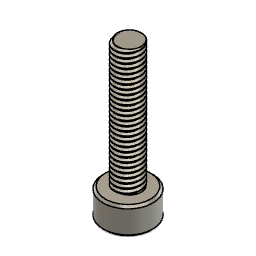
leg-test-stand-v4 (Autodesk Fusion 360 archive; units mm, degrees)
design "Cub Head Screw HEX (M3, 14mm)"
Autodesk Fusion 360 part; units mm, degrees
(part 1 of 2)
sketch "Sketch1" plane through (0, 0, 0) normal (0, 1, 0) x (1, 0, 0)
  circle A0 centre (0, 0) radius 1.5
  circle A1 centre (0, 0) radius 2.75
  line L0 (0.7217, -1.25) -> (1.4434, 0)
  line L1 (1.4434, 0) -> (0.7217, 1.25)
  line L2 (0.7217, 1.25) -> (-0.7217, 1.25)
  line L3 (-0.7217, 1.25) -> (-1.4434, 0)
  line L4 (-1.4434, 0) -> (-0.7217, -1.25)
  line L5 (-0.7217, -1.25) -> (0.7217, -1.25)
  dimension "d6" = 3
  dimension "d7" = 5.5
  dimension "d8" = 1.25
  constraint coincident A0.centre A1.centre
  constraint concentric A0 A1
  measures "d6" diameter of A0
  measures "d7" diameter of A1
  measures "d8" distance of A0.centre L5
extrude "Extrude1" add sketch "Sketch1" along normal blind 3 contours A0 | A1 | L0 L1 L2 L3 L4 L5
extrude "Extrude2" add sketch "Sketch1" along normal blind 17 contours A0 | L0 L1 L2 L3 L4 L5
extrude "Extrude3" cut sketch "Sketch1" along normal blind 1.5 contours L0 L1 L2 L3 L4 L5
thread "Thread1" "ISO Metric profile 3.0 M3x0.5 6g" major diameter 2.927 minor diameter 2.3555 pitch 0.5 angle 60 modelled right hand crest width 0.0713 on face at (1.4925, 7.6667, -0.1494) crest through (1.4635, 2.875, 0)
chamfer "Chamfer2" distance 0.25 angle 45 1 edges at (-2.5639, 3, 0.9944) 1 faces at (-0.0685, 0, 1.7474)
equation "Thread_Diameter = 3 mm"
equation "Thread_Length = 14 mm"
equation "Head_Diameter = 5.5 mm"
equation "Head_Height = 3 mm"
equation "Hex_Size = 2.5 mm"
equation "d6 = Thread_Diameter"
equation "d7 = Head_Diameter"
equation "d8 = Hex_Size / 2"
equation "d9 = Head_Height"
equation "d11 = Head_Height + Thread_Length"
equation "d13 = Head_Height / 2"

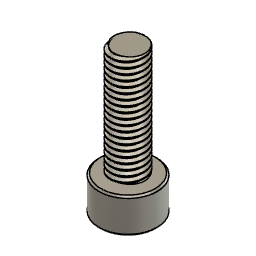
design "Cub Head Screw HEX (M5, 16mm)"
Autodesk Fusion 360 part; units mm, degrees
sketch "Sketch1" plane through (0, 0, 0) normal (0, 1, 0) x (1, 0, 0)
  circle A0 centre (0, 0) radius 2.5
  circle A1 centre (0, 0) radius 4.2
  line L0 (1.1547, -2) -> (2.3094, 0)
  line L1 (2.3094, 0) -> (1.1547, 2)
  line L2 (1.1547, 2) -> (-1.1547, 2)
  line L3 (-1.1547, 2) -> (-2.3094, 0)
  line L4 (-2.3094, 0) -> (-1.1547, -2)
  line L5 (-1.1547, -2) -> (1.1547, -2)
  dimension "d6" = 5
  dimension "d7" = 8.4
  dimension "d8" = 2
  constraint coincident A0.centre A1.centre
  constraint concentric A0 A1
  measures "d6" diameter of A0
  measures "d7" diameter of A1
  measures "d8" distance of A0.centre L5
extrude "Extrude1" add sketch "Sketch1" along normal blind 5 contours A0 | A1 | L0 L1 L2 L3 L4 L5
extrude "Extrude2" add sketch "Sketch1" along normal blind 21 contours A0 | L0 L1 L2 L3 L4 L5
extrude "Extrude3" cut sketch "Sketch1" along normal blind 2.5 contours L0 L1 L2 L3 L4 L5
thread "Thread1" "ISO Metric profile 5.0 M5x0.8 6g" major diameter 4.901 minor diameter 3.9895 pitch 0.8 angle 60 modelled right hand crest width 0.1157 on face at (2.4876, 10.3333, -0.2489) crest through (2.4505, 4.8, 0)
chamfer "Chamfer2" distance 0.25 angle 45 1 edges at (-3.9158, 5, 1.5188) 1 faces at (-0.1046, 0, 2.7294)
equation "Thread_Diameter = 5 mm"
equation "Thread_Length = 16 mm"
equation "Head_Diameter = 8.4 mm"
equation "Head_Height = 5 mm"
equation "Hex_Size = 4 mm"
equation "d6 = Thread_Diameter"
equation "d7 = Head_Diameter"
equation "d8 = Hex_Size / 2"
equation "d9 = Head_Height"
equation "d11 = Head_Height + Thread_Length"
equation "d13 = Head_Height / 2"

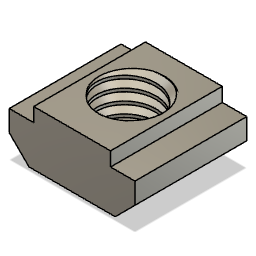
design "T-Nut (M5)"
Autodesk Fusion 360 part; units mm, degrees
sketch "Sketch1" plane through (0, 0, 0) normal (0, 0, 1) x (1, 0, 0)
  line L0 (0, 0) -> (4.5, 0)
  line L1 (4.5, 0) -> (4.5, -1.5)
  line L2 (4.5, -1.5) -> (3.0858, -2.9142)
  line L3 (4.5, -1.5) -> (6.5, -1.5) construction
  line L4 (0, 0) -> (-4.5, 0)
  line L5 (-4.5, 0) -> (-4.5, -1.5)
  line L6 (-4.5, -1.5) -> (-3.0858, -2.9142)
  line L7 (-3.0858, -2.9142) -> (3.0858, -2.9142)
  line L8 (0, 0) -> (2.75, 0)
  line L9 (2.75, 0) -> (2.75, 1)
  line L10 (0, 0) -> (-2.75, 0)
  line L11 (-2.75, 0) -> (-2.75, 1)
  line L12 (-2.75, 1) -> (2.75, 1)
  dimension "d1" = 4.5
  dimension "d2" = 1.5
  dimension "d3" = 135
  dimension "d4" = 2
  dimension "d5" = 135
  dimension "d6" = 4.5
  dimension "d7" = 1.5
  dimension "d8" = 2
  dimension "d9" = 2.75
  dimension "d10" = 1
  dimension "d11" = 2.75
  dimension "d12" = 1
  constraint coincident L0.start L4.start
  constraint horizontal L0
  constraint perpendicular L0 L1
  constraint horizontal L3
  constraint parallel L0 L4
  constraint perpendicular L0 L5
  constraint parallel L0 L8
  constraint perpendicular L8 L9
  constraint parallel L4 L10
  constraint perpendicular L4 L11
  measures "d1" distance of L0.start L0.end
  measures "d2" distance of L0.end L1.end
  measures "d3" angle of L2 L3
  measures "d4" distance of L1.end L2.end
  measures "d5" angle of L5 L6
  measures "d6" distance of L0.start L4.end
  measures "d7" distance of L4.end L5.end
  measures "d8" distance of L5.end L6.end
  measures "d9" distance of L0.start L8.end
  measures "d10" distance of L8.end L9.end
  measures "d11" distance of L0.start L10.end
  measures "d12" distance of L10.end L11.end
extrude "Extrude1" add sketch "Sketch1" along normal mid plane 8
sketch "Sketch2" plane through (0, 1, 0) normal (0, 1, 0) x (-1, 0, 0)
  line L0 (2.75, -4) -> (2.75, 4)
  line L1 (2.75, 4) -> (-2.75, 4)
  line L2 (-2.75, 4) -> (-2.75, -4)
  line L3 (-2.75, -4) -> (2.75, -4)
  circle A0 centre (0, 0) radius 2.5
  dimension "d15" = 5
  constraint coincident A0.centre origin
  measures "d15" diameter of A0
extrude "Extrude2" cut sketch "Sketch2" against normal blind 3.9142 contours A0
thread "Thread1" "ISO Metric profile 5.0 M5x0.8 6H" major diameter 5.12 minor diameter 4.234 pitch 0.8 angle 60 modelled right hand crest width 0.2219 on face at (-2.4876, -1.6095, -0.2489) crest through (-2.117, 0.8, 0)
equation "d5 = d3"
equation "d6 = d1"
equation "d7 = d2"
equation "d8 = d4"
equation "d11 = d9"
equation "d12 = d10"

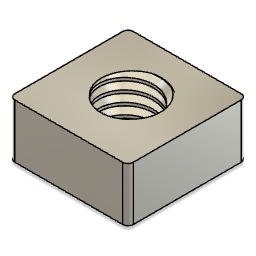
design "Square-Nut (M3)"
Autodesk Fusion 360 part; units mm, degrees
sketch "Sketch1" plane through (0, 0, 0) normal (0, 1, 0) x (1, 0, 0)
  line L0 (2.5, -2.75) -> (-2.5, -2.75)
  line L1 (-2.75, -2.5) -> (-2.75, 2.5)
  line L2 (-2.5, 2.75) -> (2.5, 2.75)
  line L3 (2.75, 2.5) -> (2.75, -2.5)
  line L4 (2.75, -2.75) -> (-2.75, 2.75) construction
  line L5 (-2.75, -2.75) -> (2.75, 2.75) construction
  circle A0 centre (0, 0) radius 1.5
  arc A1 (-2.5, 2.75) -> (-2.75, 2.5) centre (-2.5, 2.5) ccw
  arc A2 (2.75, 2.5) -> (2.5, 2.75) centre (2.5, 2.5) ccw
  arc A3 (2.5, -2.75) -> (2.75, -2.5) centre (2.5, -2.5) ccw
  arc A4 (-2.75, -2.5) -> (-2.5, -2.75) centre (-2.5, -2.5) ccw
  dimension "d1" = 5.5
  dimension "d2" = 5.5
  dimension "d3" = 3
  dimension "d4" = 0.25
  constraint horizontal L0
  constraint perpendicular L0 L1
  constraint parallel L0 L2
  constraint parallel L1 L3
  constraint coincident L4 A0.centre
  constraint coincident L5 A0.centre
  constraint coincident A0.centre origin
  constraint coincident L4.end L1
  constraint coincident L4.end L2
  constraint tangent L1 A1
  constraint tangent L2 A1
  constraint coincident L5.end L2
  constraint coincident L5.end L3
  constraint tangent L2 A2
  constraint tangent L3 A2
  constraint equal A1 A2
  constraint coincident L4.start L3
  constraint coincident L4.start L0
  constraint tangent L3 A3
  constraint tangent L0 A3
  constraint equal A1 A3
  constraint coincident L5.start L0
  constraint coincident L5.start L1
  constraint tangent L0 A4
  constraint tangent L1 A4
  constraint equal A1 A4
  measures "d1" distance of L4.end L5.end
  measures "d2" distance of L5.start L4.end
  measures "d3" diameter of A0
  measures "d4" radius of A1
extrude "Extrude1" add sketch "Sketch1" along normal blind 2.5
thread "Thread1" "ISO Metric profile 3.0 M3x0.5 6H" major diameter 3.086 minor diameter 2.529 pitch 0.5 angle 60 modelled right hand crest width 0.1368 on face at (1.4981, 1.6667, 0.0748) crest through (1.2645, 0.125, 0)
equation "d2 = d1"

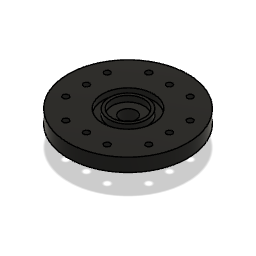
design "MG996R-servo horn"
Autodesk Fusion 360 part; units mm, degrees
sketch "Sketch1" plane through (0, 0, 0) normal (0, 1, 0) x (1, 0, 0)
  circle A0 centre (0, 0) radius 10.35
  circle A1 centre (0, 0) radius 4.4
  circle A2 centre (0, 0) radius 2.8
  circle A3 centre (0, 0) radius 3.3
  circle A4 centre (0, 0) radius 1.4
  circle A5 centre (0, 0) radius 2.6
  circle A6 centre (0, 7.2) radius 0.5
  circle A7 centre (-3.6, 7.2) radius 0.5
  circle A8 centre (3.6, 7.2) radius 0.5
  circle A9 centre (-7.2, 3.6) radius 0.5
  circle A10 centre (-7.2, 0) radius 0.5
  circle A11 centre (-7.2, -3.6) radius 0.5
  circle A12 centre (-3.6, -7.2) radius 0.5
  circle A13 centre (0, -7.2) radius 0.5
  circle A14 centre (3.6, -7.2) radius 0.5
  circle A15 centre (7.2, -3.6) radius 0.5
  circle A16 centre (7.2, 0) radius 0.5
  circle A17 centre (7.2, 3.6) radius 0.5
  dimension "d1" = 20.7
  dimension "d2" = 8.8
  dimension "d3" = 5.6
  dimension "d4" = 6.6
  dimension "d5" = 2.8
  dimension "d6" = 5.2
  dimension "d7" = 1
  dimension "d8" = 7.2
  dimension "d11" = 3.6
  dimension "d12" = 0
  dimension "d14" = 360
  constraint coincident A0.centre A1.centre
  constraint concentric A0 A1
  constraint concentric A0 A2
  constraint concentric A1 A3
  constraint concentric A1 A5
  measures "d1" diameter of A0
  measures "d2" diameter of A1
  measures "d3" diameter of A2
  measures "d4" diameter of A3
  measures "d5" diameter of A4
  measures "d6" diameter of A5
  measures "d7" diameter of A6
  measures "d8" distance of A0.centre A6.centre
extrude "Extrude1" add sketch "Sketch1" against normal blind 3.55 contours A1 | A2 | A3
extrude "Extrude4" add sketch "Sketch1" against normal blind 0.55 contours A5
extrude "Extrude2" add sketch "Sketch1" along normal blind 2.3 contours A0 | A1 | A2 | A3 | A5
extrude "Extrude3" cut sketch "Sketch1" against normal blind 1 from surface at 2.3 contours A1 | A2 | A5
equation "d8 = ( 14.4 / 2 ) * 1 mm"

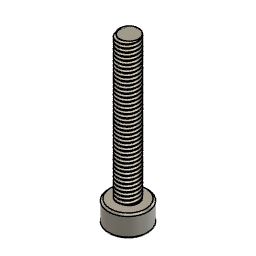
design "Cub Head Screw HEX (M3, 20mm)"
Autodesk Fusion 360 part; units mm, degrees
sketch "Sketch1" plane through (0, 0, 0) normal (0, 1, 0) x (1, 0, 0)
  circle A0 centre (0, 0) radius 1.5
  circle A1 centre (0, 0) radius 2.75
  line L0 (0.7217, -1.25) -> (1.4434, 0)
  line L1 (1.4434, 0) -> (0.7217, 1.25)
  line L2 (0.7217, 1.25) -> (-0.7217, 1.25)
  line L3 (-0.7217, 1.25) -> (-1.4434, 0)
  line L4 (-1.4434, 0) -> (-0.7217, -1.25)
  line L5 (-0.7217, -1.25) -> (0.7217, -1.25)
  dimension "d6" = 3
  dimension "d7" = 5.5
  dimension "d8" = 1.25
  constraint coincident A0.centre A1.centre
  constraint concentric A0 A1
  measures "d6" diameter of A0
  measures "d7" diameter of A1
  measures "d8" distance of A0.centre L5
extrude "Extrude1" add sketch "Sketch1" along normal blind 3 contours A0 | A1 | L0 L1 L2 L3 L4 L5
extrude "Extrude2" add sketch "Sketch1" along normal blind 23 contours A0 | L0 L1 L2 L3 L4 L5
extrude "Extrude3" cut sketch "Sketch1" along normal blind 1.5 contours L0 L1 L2 L3 L4 L5
thread "Thread1" "ISO Metric profile 3.0 M3x0.5 6g" major diameter 2.927 minor diameter 2.3555 pitch 0.5 angle 60 modelled right hand crest width 0.0713 on face at (1.4925, 9.6667, -0.1494) crest through (1.4635, 2.875, 0)
chamfer "Chamfer2" distance 0.25 angle 45 1 edges at (-2.5639, 3, 0.9944) 1 faces at (-0.0685, 0, 1.7474)
equation "Thread_Diameter = 3 mm"
equation "Thread_Length = 20 mm"
equation "Head_Diameter = 5.5 mm"
equation "Head_Height = 3 mm"
equation "Hex_Size = 2.5 mm"
equation "d6 = Thread_Diameter"
equation "d7 = Head_Diameter"
equation "d8 = Hex_Size / 2"
equation "d9 = Head_Height"
equation "d11 = Head_Height + Thread_Length"
equation "d13 = Head_Height / 2"

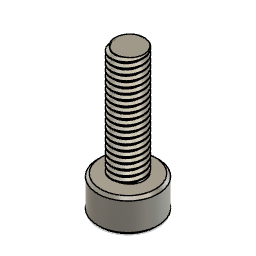
design "Cub Head Screw HEX (M3, 10mm)"
Autodesk Fusion 360 part; units mm, degrees
sketch "Sketch1" plane through (0, 0, 0) normal (0, 1, 0) x (1, 0, 0)
  circle A0 centre (0, 0) radius 1.5
  circle A1 centre (0, 0) radius 2.75
  line L0 (0.7217, -1.25) -> (1.4434, 0)
  line L1 (1.4434, 0) -> (0.7217, 1.25)
  line L2 (0.7217, 1.25) -> (-0.7217, 1.25)
  line L3 (-0.7217, 1.25) -> (-1.4434, 0)
  line L4 (-1.4434, 0) -> (-0.7217, -1.25)
  line L5 (-0.7217, -1.25) -> (0.7217, -1.25)
  dimension "d6" = 3
  dimension "d7" = 5.5
  dimension "d8" = 1.25
  constraint coincident A0.centre A1.centre
  constraint concentric A0 A1
  measures "d6" diameter of A0
  measures "d7" diameter of A1
  measures "d8" distance of A0.centre L5
extrude "Extrude1" add sketch "Sketch1" along normal blind 3 contours A0 | A1 | L0 L1 L2 L3 L4 L5
extrude "Extrude2" add sketch "Sketch1" along normal blind 13 contours A0 | L0 L1 L2 L3 L4 L5
extrude "Extrude3" cut sketch "Sketch1" along normal blind 1.5 contours L0 L1 L2 L3 L4 L5
thread "Thread1" "ISO Metric profile 3.0 M3x0.5 6g" major diameter 2.927 minor diameter 2.3555 pitch 0.5 angle 60 modelled right hand crest width 0.0713 on face at (1.4925, 6.3333, -0.1494) crest through (1.4635, 2.875, 0)
chamfer "Chamfer2" distance 0.25 angle 45 1 edges at (-2.5639, 3, 0.9944) 1 faces at (-0.0685, 0, 1.7474)
equation "Thread_Diameter = 3 mm"
equation "Thread_Length = 10 mm"
equation "Head_Diameter = 5.5 mm"
equation "Head_Height = 3 mm"
equation "Hex_Size = 2.5 mm"
equation "d6 = Thread_Diameter"
equation "d7 = Head_Diameter"
equation "d8 = Hex_Size / 2"
equation "d9 = Head_Height"
equation "d11 = Head_Height + Thread_Length"
equation "d13 = Head_Height / 2"

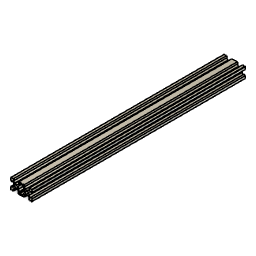
design "Extrusions-2040 (400mm)"
Autodesk Fusion 360 part; units mm, degrees
sketch "Skizze1" plane through (0, 0, 0) normal (0, 0, 1) x (1, 0, 0)
  line L0 (0, 0) -> (20, 0)
  line L1 (20, 0) -> (20, 20)
  line L2 (20, 20) -> (0, 20)
  line L3 (0, 20) -> (0, 0)
  circle A0 centre (10, 10) radius 2.5
  line L4 (0, 0) -> (6.8, 0)
  line L5 (6.8, 0) -> (13.2, 0)
  line L6 (6.8, 0) -> (13.2, 0)
  line L7 (13.2, 0) -> (13.2, 1.8)
  line L8 (13.2, 1.8) -> (6.8, 1.8)
  line L9 (6.8, 1.8) -> (6.8, 0)
  line L10 (0, 0) -> (0, 6.8)
  line L11 (0, 20) -> (6.8, 20)
  line L12 (20, 0) -> (20, 6.8)
  line L13 (0, 6.8) -> (1.8, 6.8)
  line L14 (1.8, 6.8) -> (1.8, 13.2)
  line L15 (1.8, 13.2) -> (0, 13.2)
  line L16 (0, 13.2) -> (0, 6.8)
  line L17 (6.8, 20) -> (13.2, 20)
  line L18 (13.2, 20) -> (13.2, 18.2)
  line L19 (13.2, 18.2) -> (6.8, 18.2)
  line L20 (6.8, 18.2) -> (6.8, 20)
  line L21 (20, 6.8) -> (18.2, 6.8)
  line L22 (18.2, 6.8) -> (18.2, 13.2)
  line L23 (18.2, 13.2) -> (20, 13.2)
  line L24 (20, 13.2) -> (20, 6.8)
  line L25 (10, 1.8) -> (15, 1.8)
  line L26 (15, 1.8) -> (15, 3.6)
  line L27 (15, 3.6) -> (10, 3.6)
  line L28 (10, 3.6) -> (10, 1.8)
  line L29 (15, 1.8) -> (5, 1.8)
  line L30 (5, 1.8) -> (5, 3.6)
  line L31 (5, 3.6) -> (15, 3.6)
  line L32 (15, 3.6) -> (15, 1.8)
  line L33 (10, 18.2) -> (15, 18.2)
  line L34 (15, 18.2) -> (15, 16.4)
  line L35 (15, 16.4) -> (10, 16.4)
  line L36 (10, 16.4) -> (10, 18.2)
  line L37 (15, 16.4) -> (5, 16.4)
  line L38 (5, 16.4) -> (5, 18.2)
  line L39 (5, 18.2) -> (15, 18.2)
  line L40 (15, 18.2) -> (15, 16.4)
  line L41 (1.8, 10) -> (3.6, 10)
  line L42 (3.6, 10) -> (3.6, 5)
  line L43 (3.6, 5) -> (1.8, 5)
  line L44 (1.8, 5) -> (1.8, 10)
  line L45 (3.6, 5) -> (1.8, 5)
  line L46 (1.8, 5) -> (1.8, 15)
  line L47 (1.8, 15) -> (3.6, 15)
  line L48 (3.6, 15) -> (3.6, 5)
  line L49 (18.2, 10) -> (16.4, 10)
  line L50 (16.4, 10) -> (16.4, 15)
  line L51 (16.4, 15) -> (18.2, 15)
  line L52 (18.2, 15) -> (18.2, 10)
  line L53 (16.4, 15) -> (18.2, 15)
  line L54 (18.2, 15) -> (18.2, 5)
  line L55 (18.2, 5) -> (16.4, 5)
  line L56 (16.4, 5) -> (16.4, 15)
  line L57 (6, 6) -> (14, 6)
  line L58 (14, 6) -> (14, 14)
  line L59 (14, 14) -> (6, 14)
  line L60 (6, 14) -> (6, 6)
  line L61 (5, 3.6) -> (7.4, 6)
  line L62 (5, 3.6) -> (8.3941, 3.6) construction
  line L63 (3.6, 5) -> (6, 7.4)
  line L64 (15, 3.6) -> (12.6, 6)
  line L65 (16.4, 5) -> (14, 7.4)
  line L66 (16.4, 15) -> (14, 12.6)
  line L67 (15, 16.4) -> (12.6, 14)
  line L68 (3.6, 15) -> (6, 12.6)
  line L69 (5, 16.4) -> (7.4, 14)
  line L70 (6.8, 1.8) -> (5, 0)
  line L71 (18.2, 5) -> (20.7456, 5) construction
  line L72 (18.2, 6.8) -> (20, 5)
  line L73 (18.2, 13.2) -> (20, 15)
  line L74 (18.2, 13.2) -> (20.7456, 13.2) construction
  line L75 (6.8, 18.2) -> (5, 20)
  line L76 (13.2, 18.2) -> (15, 20)
  line L77 (1.8, 13.2) -> (0, 15)
  line L78 (1.8, 6.8) -> (0, 5)
  line L79 (13.2, 1.8) -> (15, 0)
  dimension "d1" = 5
  dimension "d2" = 6.8
  dimension "d3" = 6.4
  dimension "d4" = 1.8
  dimension "d5" = 6.8
  dimension "d6" = 6.8
  dimension "d7" = 6.8
  dimension "d8" = 1.8
  dimension "d9" = 6.4
  dimension "d10" = 1.8
  dimension "d11" = 1.8
  dimension "d12" = 5
  dimension "d13" = 1.8
  dimension "d14" = 10
  dimension "d15" = 1.8
  dimension "d16" = 1.8
  dimension "d17" = 10
  dimension "d18" = 1.8
  dimension "d19" = 10
  dimension "d20" = 45
  dimension "d22" = 45
  constraint horizontal L0
  constraint vertical L1
  constraint horizontal L2
  constraint vertical L3
  constraint coincident L0.start L3.end
  constraint perpendicular L3 L4
  constraint parallel L0 L5
  constraint horizontal L6
  constraint vertical L7
  constraint horizontal L8
  constraint vertical L9
  constraint perpendicular L4 L10
  constraint perpendicular L3 L11
  constraint perpendicular L11 L12
  constraint horizontal L13
  constraint vertical L14
  constraint horizontal L15
  constraint vertical L16
  constraint horizontal L17
  constraint vertical L18
  constraint horizontal L19
  constraint vertical L20
  constraint horizontal L21
  constraint vertical L22
  constraint horizontal L23
  constraint vertical L24
  constraint horizontal L25
  constraint vertical L26
  constraint horizontal L27
  constraint vertical L28
  constraint midpoint L8 L25.start
  constraint horizontal L29
  constraint vertical L30
  constraint horizontal L31
  constraint vertical L32
  constraint horizontal L33
  constraint vertical L34
  constraint horizontal L35
  constraint vertical L36
  constraint midpoint L19 L33.start
  constraint horizontal L37
  constraint vertical L38
  constraint horizontal L39
  constraint vertical L40
  constraint horizontal L41
  constraint vertical L42
  constraint horizontal L43
  constraint vertical L44
  constraint midpoint L14 L41.start
  constraint horizontal L45
  constraint vertical L46
  constraint horizontal L47
  constraint vertical L48
  constraint horizontal L49
  constraint vertical L50
  constraint horizontal L51
  constraint vertical L52
  constraint midpoint L22 L49.start
  constraint horizontal L53
  constraint vertical L54
  constraint horizontal L55
  constraint vertical L56
  constraint horizontal L57
  constraint vertical L58
  constraint horizontal L59
  constraint vertical L60
  constraint horizontal L62
  constraint coincident L57 L61.end
  constraint coincident L60 L63.end
  constraint parallel L61 L63
  constraint coincident L57 L64.end
  constraint perpendicular L63 L64
  constraint coincident L58 L65.end
  constraint parallel L64 L65
  constraint coincident L58 L66.end
  constraint perpendicular L65 L66
  constraint coincident L59 L67.end
  constraint parallel L66 L67
  constraint coincident L60 L68.end
  constraint perpendicular L67 L68
  constraint coincident L59 L69.end
  constraint parallel L68 L69
  constraint coincident L0 L70.end
  constraint horizontal L71
  constraint coincident L12 L72.end
  constraint horizontal L74
  constraint coincident L1 L73.end
  constraint coincident L2 L75.end
  constraint coincident L2 L76.end
  constraint perpendicular L75 L76
  constraint coincident L3 L77.end
  constraint perpendicular L76 L77
  constraint coincident L10 L78.end
  constraint coincident L0 L79.end
  measures "d1" diameter of A0
  measures "d2" distance of L0.start L4.end
  measures "d3" distance of L4.end L5.end
  measures "d4" distance of L4.end L8.end
  measures "d5" distance of L0.start L10.end
  measures "d6" distance of L2.end L11.end
  measures "d7" distance of L0.end L12.end
  measures "d8" distance of L10.end L13.end
  measures "d9" distance of L10.end L15.end
  measures "d10" distance of L11.end L19.end
  measures "d11" distance of L12.end L21.end
  measures "d12" distance of L25.start L25.end
  measures "d13" distance of L25.start L27.end
  measures "d14" distance of L25.end L29.end
  measures "d15" distance of L33.start L35.end
  measures "d16" distance of L41.start L41.end
  measures "d17" distance of L42.end L47.end
  measures "d18" distance of L49.start L49.end
  measures "d19" distance of L50.end L55.end
  measures "d20" angle of L61 L62
  measures "d22" angle of L73 L74
extrude "Extrusion1" add sketch "Skizze1" along normal mid plane 400 contours L0 L3 L4 L10 L29 L30 L43 L44 L45 L46 L57 L60 L61 L63 L70 L78 | L0 L1 L12 L25 L26 L29 L32 L54 L55 L57 L58 L64 L65 L72 L79 | L2 L3 L11 L38 L39 L46 L47 L59 L60 L68 L69 L75 L77 | L57 L58 L59 L60 | L1 L2 L33 L34 L39 L40 L51 L52 L53 L54 L58 L59 L66 L67 L73 L76 makes body 1
copy_body "Körper kopieren/einfügen1" bodies 1 makes body 2
move_body "Verschieben1" bodies 2 to x (1, 0, 0) y (0, 1, 0) z (0, 0, 1) at (25, 0, 0)
copy_body "Körper kopieren/einfügen2" bodies 2 makes body 3
move_body "Verschieben2" bodies 3 to x (1, 0, 0) y (0, 1, 0) z (0, 0, 1) at (0, 20, 0)
combine "Kombinieren1" operation add target body 2 tool bodies 3
sketch "Skizze2" plane through (0, 0, 200) normal (0, 0, 1) x (1, 0, 0)
  line L0 (40, 20) -> (38.2, 18.2)
  line L1 (38.2, 18.2) -> (40, 18.2)
  line L2 (40, 18.2) -> (40, 16.4)
  line L3 (40, 16.4) -> (37.6, 14)
  line L4 (37.6, 14) -> (32.4, 14)
  line L5 (32.4, 14) -> (30, 16.4)
  line L6 (30, 16.4) -> (30, 18.2)
  line L7 (30, 18.2) -> (31.8, 18.2)
  line L8 (31.8, 18.2) -> (30, 20)
  line L9 (30, 20) -> (31.8, 21.8)
  line L10 (31.8, 21.8) -> (30, 21.8)
  line L11 (30, 21.8) -> (30, 23.6)
  line L12 (30, 23.6) -> (32.4, 26)
  line L13 (32.4, 26) -> (37.6, 26)
  line L14 (37.6, 26) -> (40, 23.6)
  line L15 (40, 23.6) -> (40, 21.8)
  line L16 (40, 21.8) -> (38.2, 21.8)
  line L17 (38.2, 21.8) -> (40, 20)
  circle A0 centre (35, 30) radius 2.5
  circle A1 centre (35, 10) radius 2.5
  line L18 (45, 15) -> (45, 25)
  line L19 (45, 25) -> (43.2, 26.8)
  line L20 (43.2, 26.8) -> (43.2, 25)
  line L21 (43.2, 25) -> (41.4, 25)
  line L22 (41.4, 25) -> (39, 27.4)
  line L23 (39, 27.4) -> (39, 32.6)
  line L24 (39, 32.6) -> (41.4, 35)
  line L25 (41.4, 35) -> (43.2, 35)
  line L26 (43.2, 35) -> (43.2, 33.2)
  line L27 (43.2, 33.2) -> (45, 35)
  line L28 (45, 35) -> (45, 40)
  line L29 (45, 40) -> (40, 40)
  line L30 (40, 40) -> (38.2, 38.2)
  line L31 (38.2, 38.2) -> (40, 38.2)
  line L32 (40, 38.2) -> (40, 36.4)
  line L33 (40, 36.4) -> (37.6, 34)
  line L34 (37.6, 34) -> (32.4, 34)
  line L35 (32.4, 34) -> (30, 36.4)
  line L36 (30, 36.4) -> (30, 38.2)
  line L37 (30, 38.2) -> (31.8, 38.2)
  line L38 (31.8, 38.2) -> (30, 40)
  line L39 (30, 40) -> (25, 40)
  line L40 (25, 40) -> (25, 35)
  line L41 (25, 35) -> (26.8, 33.2)
  line L42 (26.8, 33.2) -> (26.8, 35)
  line L43 (26.8, 35) -> (28.6, 35)
  line L44 (28.6, 35) -> (31, 32.6)
  line L45 (31, 32.6) -> (31, 27.4)
  line L46 (31, 27.4) -> (28.6, 25)
  line L47 (28.6, 25) -> (26.8, 25)
  line L48 (26.8, 25) -> (26.8, 26.8)
  line L49 (26.8, 26.8) -> (25, 25)
  line L50 (25, 25) -> (25, 15)
  line L51 (25, 15) -> (26.8, 13.2)
  line L52 (26.8, 13.2) -> (26.8, 15)
  line L53 (26.8, 15) -> (28.6, 15)
  line L54 (28.6, 15) -> (31, 12.6)
  line L55 (31, 12.6) -> (31, 7.4)
  line L56 (31, 7.4) -> (28.6, 5)
  line L57 (28.6, 5) -> (26.8, 5)
  line L58 (26.8, 5) -> (26.8, 6.8)
  line L59 (26.8, 6.8) -> (25, 5)
  line L60 (25, 5) -> (25, 0)
  line L61 (25, 0) -> (30, 0)
  line L62 (30, 0) -> (31.8, 1.8)
  line L63 (31.8, 1.8) -> (30, 1.8)
  line L64 (30, 1.8) -> (30, 3.6)
  line L65 (30, 3.6) -> (32.4, 6)
  line L66 (32.4, 6) -> (37.6, 6)
  line L67 (37.6, 6) -> (40, 3.6)
  line L68 (40, 3.6) -> (40, 1.8)
  line L69 (40, 1.8) -> (38.2, 1.8)
  line L70 (38.2, 1.8) -> (40, 0)
  line L71 (40, 0) -> (45, 0)
  line L72 (45, 0) -> (45, 5)
  line L73 (45, 5) -> (43.2, 6.8)
  line L74 (43.2, 6.8) -> (43.2, 5)
  line L75 (43.2, 5) -> (41.4, 5)
  line L76 (41.4, 5) -> (39, 7.4)
  line L77 (39, 7.4) -> (39, 12.6)
  line L78 (39, 12.6) -> (41.4, 15)
  line L79 (41.4, 15) -> (43.2, 15)
  line L80 (43.2, 15) -> (43.2, 13.2)
  line L81 (43.2, 13.2) -> (45, 15)
  line L82 (26.8, 15) -> (26.8, 16.98)
  line L83 (26.8, 25) -> (26.8, 23.02)
  line L84 (26.8, 16.98) -> (28.8, 16.98)
  line L85 (28.8, 16.98) -> (28.8, 23.02)
  line L86 (28.8, 23.02) -> (26.8, 23.02)
  line L87 (26.8, 23.02) -> (26.8, 16.98)
  dimension "d25" = 1.98
  dimension "d26" = 1.98
  dimension "d27" = 2
  constraint coincident L52.end L53.start
  constraint perpendicular L53 L82
  constraint coincident L47.end L48.start
  constraint perpendicular L47 L83
  constraint horizontal L84
  constraint vertical L85
  constraint horizontal L86
  constraint vertical L87
  measures "d25" distance of L52.end L82.end
  measures "d26" distance of L47.end L83.end
  measures "d27" distance of L82.end L84.end
extrude "Extrusion2" cut sketch "Skizze2" against normal blind 126 contours L84 L85 L86 L87 bodies 2
sketch "Skizze3" plane through (0, 0, 200) normal (0, 0, 1) x (1, 0, 0)
  line L0 (28.8, 16.98) -> (26.8, 16.98)
  line L1 (26.8, 16.98) -> (26.8, 23.02)
  line L2 (26.8, 23.02) -> (28.8, 23.02)
  line L3 (28.8, 23.02) -> (28.8, 16.98)
  line L4 (40, 20) -> (38.2, 18.2)
  line L5 (38.2, 18.2) -> (40, 18.2)
  line L6 (40, 18.2) -> (40, 16.4)
  line L7 (40, 16.4) -> (37.6, 14)
  line L8 (37.6, 14) -> (32.4, 14)
  line L9 (32.4, 14) -> (30, 16.4)
  line L10 (30, 16.4) -> (30, 18.2)
  line L11 (30, 18.2) -> (31.8, 18.2)
  line L12 (31.8, 18.2) -> (30, 20)
  line L13 (30, 20) -> (31.8, 21.8)
  line L14 (31.8, 21.8) -> (30, 21.8)
  line L15 (30, 21.8) -> (30, 23.6)
  line L16 (30, 23.6) -> (32.4, 26)
  line L17 (32.4, 26) -> (37.6, 26)
  line L18 (37.6, 26) -> (40, 23.6)
  line L19 (40, 23.6) -> (40, 21.8)
  line L20 (40, 21.8) -> (38.2, 21.8)
  line L21 (38.2, 21.8) -> (40, 20)
  circle A0 centre (35, 30) radius 2.5
  circle A1 centre (35, 10) radius 2.5
  line L22 (45, 15) -> (45, 25)
  line L23 (45, 25) -> (43.2, 26.8)
  line L24 (43.2, 26.8) -> (43.2, 25)
  line L25 (43.2, 25) -> (41.4, 25)
  line L26 (41.4, 25) -> (39, 27.4)
  line L27 (39, 27.4) -> (39, 32.6)
  line L28 (39, 32.6) -> (41.4, 35)
  line L29 (41.4, 35) -> (43.2, 35)
  line L30 (43.2, 35) -> (43.2, 33.2)
  line L31 (43.2, 33.2) -> (45, 35)
  line L32 (45, 35) -> (45, 40)
  line L33 (45, 40) -> (40, 40)
  line L34 (40, 40) -> (38.2, 38.2)
  line L35 (38.2, 38.2) -> (40, 38.2)
  line L36 (40, 38.2) -> (40, 36.4)
  line L37 (40, 36.4) -> (37.6, 34)
  line L38 (37.6, 34) -> (32.4, 34)
  line L39 (32.4, 34) -> (30, 36.4)
  line L40 (30, 36.4) -> (30, 38.2)
  line L41 (30, 38.2) -> (31.8, 38.2)
  line L42 (31.8, 38.2) -> (30, 40)
  line L43 (30, 40) -> (25, 40)
  line L44 (25, 40) -> (25, 35)
  line L45 (25, 35) -> (26.8, 33.2)
  line L46 (26.8, 33.2) -> (26.8, 35)
  line L47 (26.8, 35) -> (28.6, 35)
  line L48 (28.6, 35) -> (31, 32.6)
  line L49 (31, 32.6) -> (31, 27.4)
  line L50 (31, 27.4) -> (28.6, 25)
  line L51 (28.6, 25) -> (26.8, 25)
  line L52 (26.8, 25) -> (26.8, 26.8)
  line L53 (26.8, 26.8) -> (25, 25)
  line L54 (25, 25) -> (25, 15)
  line L55 (25, 15) -> (26.8, 13.2)
  line L56 (26.8, 13.2) -> (26.8, 15)
  line L57 (26.8, 15) -> (28.6, 15)
  line L58 (28.6, 15) -> (31, 12.6)
  line L59 (31, 12.6) -> (31, 7.4)
  line L60 (31, 7.4) -> (28.6, 5)
  line L61 (28.6, 5) -> (26.8, 5)
  line L62 (26.8, 5) -> (26.8, 6.8)
  line L63 (26.8, 6.8) -> (25, 5)
  line L64 (25, 5) -> (25, 0)
  line L65 (25, 0) -> (30, 0)
  line L66 (30, 0) -> (31.8, 1.8)
  line L67 (31.8, 1.8) -> (30, 1.8)
  line L68 (30, 1.8) -> (30, 3.6)
  line L69 (30, 3.6) -> (32.4, 6)
  line L70 (32.4, 6) -> (37.6, 6)
  line L71 (37.6, 6) -> (40, 3.6)
  line L72 (40, 3.6) -> (40, 1.8)
  line L73 (40, 1.8) -> (38.2, 1.8)
  line L74 (38.2, 1.8) -> (40, 0)
  line L75 (40, 0) -> (45, 0)
  line L76 (45, 0) -> (45, 5)
  line L77 (45, 5) -> (43.2, 6.8)
  line L78 (43.2, 6.8) -> (43.2, 5)
  line L79 (43.2, 5) -> (41.4, 5)
  line L80 (41.4, 5) -> (39, 7.4)
  line L81 (39, 7.4) -> (39, 12.6)
  line L82 (39, 12.6) -> (41.4, 15)
  line L83 (41.4, 15) -> (43.2, 15)
  line L84 (43.2, 15) -> (43.2, 13.2)
  line L85 (43.2, 13.2) -> (45, 15)
extrude "Extrusion3" add sketch "Skizze3" against normal blind 100 contours L0 L1 L2 L3 bodies 2
sketch "Skizze4" plane through (0, 0, 200) normal (0, 0, 1) x (1, 0, 0)
  line L0 (40, 20) -> (38.2, 18.2)
  line L1 (38.2, 18.2) -> (40, 18.2)
  line L2 (40, 18.2) -> (40, 16.4)
  line L3 (40, 16.4) -> (37.6, 14)
  line L4 (37.6, 14) -> (32.4, 14)
  line L5 (32.4, 14) -> (30, 16.4)
  line L6 (30, 16.4) -> (30, 18.2)
  line L7 (30, 18.2) -> (31.8, 18.2)
  line L8 (31.8, 18.2) -> (30, 20)
  line L9 (30, 20) -> (31.8, 21.8)
  line L10 (31.8, 21.8) -> (30, 21.8)
  line L11 (30, 21.8) -> (30, 23.6)
  line L12 (30, 23.6) -> (32.4, 26)
  line L13 (32.4, 26) -> (37.6, 26)
  line L14 (37.6, 26) -> (40, 23.6)
  line L15 (40, 23.6) -> (40, 21.8)
  line L16 (40, 21.8) -> (38.2, 21.8)
  line L17 (38.2, 21.8) -> (40, 20)
  circle A0 centre (35, 30) radius 2.5
  circle A1 centre (35, 10) radius 2.5
  line L18 (45, 15) -> (45, 25)
  line L19 (45, 25) -> (43.2, 26.8)
  line L20 (43.2, 26.8) -> (43.2, 25)
  line L21 (43.2, 25) -> (41.4, 25)
  line L22 (41.4, 25) -> (39, 27.4)
  line L23 (39, 27.4) -> (39, 32.6)
  line L24 (39, 32.6) -> (41.4, 35)
  line L25 (41.4, 35) -> (43.2, 35)
  line L26 (43.2, 35) -> (43.2, 33.2)
  line L27 (43.2, 33.2) -> (45, 35)
  line L28 (45, 35) -> (45, 40)
  line L29 (45, 40) -> (40, 40)
  line L30 (40, 40) -> (38.2, 38.2)
  line L31 (38.2, 38.2) -> (40, 38.2)
  line L32 (40, 38.2) -> (40, 36.4)
  line L33 (40, 36.4) -> (37.6, 34)
  line L34 (37.6, 34) -> (32.4, 34)
  line L35 (32.4, 34) -> (30, 36.4)
  line L36 (30, 36.4) -> (30, 38.2)
  line L37 (30, 38.2) -> (31.8, 38.2)
  line L38 (31.8, 38.2) -> (30, 40)
  line L39 (30, 40) -> (25, 40)
  line L40 (25, 40) -> (25, 35)
  line L41 (25, 35) -> (26.8, 33.2)
  line L42 (26.8, 33.2) -> (26.8, 35)
  line L43 (26.8, 35) -> (28.6, 35)
  line L44 (28.6, 35) -> (31, 32.6)
  line L45 (31, 32.6) -> (31, 27.4)
  line L46 (31, 27.4) -> (28.6, 25)
  line L47 (28.6, 25) -> (26.8, 25)
  line L48 (26.8, 25) -> (26.8, 26.8)
  line L49 (26.8, 26.8) -> (25, 25)
  line L50 (25, 25) -> (25, 15)
  line L51 (25, 15) -> (26.8, 13.2)
  line L52 (26.8, 13.2) -> (26.8, 15)
  line L53 (26.8, 15) -> (28.6, 15)
  line L54 (28.6, 15) -> (31, 12.6)
  line L55 (31, 12.6) -> (31, 7.4)
  line L56 (31, 7.4) -> (28.6, 5)
  line L57 (28.6, 5) -> (26.8, 5)
  line L58 (26.8, 5) -> (26.8, 6.8)
  line L59 (26.8, 6.8) -> (25, 5)
  line L60 (25, 5) -> (25, 0)
  line L61 (25, 0) -> (30, 0)
  line L62 (30, 0) -> (31.8, 1.8)
  line L63 (31.8, 1.8) -> (30, 1.8)
  line L64 (30, 1.8) -> (30, 3.6)
  line L65 (30, 3.6) -> (32.4, 6)
  line L66 (32.4, 6) -> (37.6, 6)
  line L67 (37.6, 6) -> (40, 3.6)
  line L68 (40, 3.6) -> (40, 1.8)
  line L69 (40, 1.8) -> (38.2, 1.8)
  line L70 (38.2, 1.8) -> (40, 0)
  line L71 (40, 0) -> (45, 0)
  line L72 (45, 0) -> (45, 5)
  line L73 (45, 5) -> (43.2, 6.8)
  line L74 (43.2, 6.8) -> (43.2, 5)
  line L75 (43.2, 5) -> (41.4, 5)
  line L76 (41.4, 5) -> (39, 7.4)
  line L77 (39, 7.4) -> (39, 12.6)
  line L78 (39, 12.6) -> (41.4, 15)
  line L79 (41.4, 15) -> (43.2, 15)
  line L80 (43.2, 15) -> (43.2, 13.2)
  line L81 (43.2, 13.2) -> (45, 15)
  line L82 (26.8, 15) -> (26.8, 17)
  line L83 (26.8, 25) -> (26.8, 23)
  line L84 (26.8, 17) -> (29.5, 17)
  line L85 (29.5, 17) -> (29.5, 23)
  line L86 (29.5, 23) -> (26.8, 23)
  line L87 (26.8, 23) -> (26.8, 17)
  line L88 (30, 16.4) -> (29.4, 17)
  line L89 (30, 23.6) -> (29.4, 23)
  line L90 (43.2, 15) -> (43.2, 17)
  line L91 (43.2, 17) -> (40.4816, 17)
  line L92 (40.4816, 17) -> (40.4816, 23)
  line L93 (40.4816, 23) -> (43.2, 23)
  line L94 (43.2, 23) -> (43.2, 17)
  line L95 (40, 16.4) -> (40.6, 17)
  line L96 (40, 23.6) -> (40.6, 23)
  dimension "d32" = 2
  dimension "d33" = 2
  constraint coincident L52.end L53.start
  constraint perpendicular L53 L82
  constraint coincident L47.end L48.start
  constraint perpendicular L47 L83
  constraint horizontal L84
  constraint vertical L85
  constraint horizontal L86
  constraint vertical L87
  constraint coincident L5.end L6.start
  constraint coincident L84 L88.end
  constraint parallel L5 L88
  constraint coincident L11.end L12.start
  constraint coincident L86 L89.end
  constraint perpendicular L88 L89
  constraint coincident L79.end L80.start
  constraint perpendicular L79 L90
  constraint horizontal L91
  constraint vertical L92
  constraint horizontal L93
  constraint vertical L94
  constraint coincident L2.end L3.start
  constraint coincident L91 L95.end
  constraint parallel L3 L95
  constraint coincident L14.end L15.start
  constraint coincident L93 L96.end
  constraint perpendicular L95 L96
  measures "d32" distance of L52.end L82.end
  measures "d33" distance of L47.end L83.end
extrude "Extrusion4" cut sketch "Skizze4" against normal blind 115 contours L0 L1 L2 L15 L16 L17 L91 L92 L93 L95 L96 | L91 L92 L93 L94 | L6 L7 L8 L9 L10 L11 L84 L85 L86 L88 L89 | L84 L85 L86 L87 bodies 2
copy_body "Körper kopieren/einfügen3" bodies 2 makes body 4
move_body "Verschieben3" bodies 4 to x (1, 0, 0) y (0, 1, 0) z (0, 0, 1) at (25, 0, 0)
copy_body "Körper kopieren/einfügen4" bodies 4 makes body 5
move_body "Verschieben4" bodies 5 to x (1, 0, 0) y (0, 1, 0) z (0, 0, 1) at (0, 20, 0)
combine "Kombinieren2" operation add target body 4 tool bodies 5
copy_body "Körper kopieren/einfügen5" bodies 2 makes body 6
move_body "Verschieben5" bodies 6 to x (1, 0, 0) y (0, 1, 0) z (0, 0, 1) at (50, 0, 0)
copy_body "Körper kopieren/einfügen6" bodies 6 makes body 7
move_body "Verschieben6" bodies 7 to x (1, 0, 0) y (0, 1, 0) z (0, 0, 1) at (0, 40, 0)
combine "Kombinieren3" operation add target body 6 tool bodies 7
sketch "Skizze5" plane through (0, 0, 200) normal (0, 0, 1) x (1, 0, 0)
  line L0 (50, 45) -> (50, 35)
  line L1 (50, 35) -> (51.8, 33.2)
  line L2 (51.8, 33.2) -> (51.8, 35)
  line L3 (51.8, 35) -> (53.6, 35)
  line L4 (53.6, 35) -> (56, 32.6)
  line L5 (56, 32.6) -> (56, 27.4)
  line L6 (56, 27.4) -> (53.6, 25)
  line L7 (53.6, 25) -> (51.8, 25)
  line L8 (51.8, 25) -> (51.8, 26.8)
  line L9 (51.8, 26.8) -> (50, 25)
  line L10 (50, 25) -> (50, 15)
  line L11 (50, 15) -> (51.8, 13.2)
  line L12 (51.8, 13.2) -> (51.8, 15)
  line L13 (51.8, 15) -> (53.6, 15)
  line L14 (53.6, 15) -> (56, 12.6)
  line L15 (56, 12.6) -> (56, 7.4)
  line L16 (56, 7.4) -> (53.6, 5)
  line L17 (53.6, 5) -> (51.8, 5)
  line L18 (51.8, 5) -> (51.8, 6.8)
  line L19 (51.8, 6.8) -> (50, 5)
  line L20 (50, 5) -> (50, 0)
  line L21 (50, 0) -> (55, 0)
  line L22 (55, 0) -> (56.8, 1.8)
  line L23 (56.8, 1.8) -> (55, 1.8)
  line L24 (55, 1.8) -> (55, 3.6)
  line L25 (55, 3.6) -> (57.4, 6)
  line L26 (57.4, 6) -> (62.6, 6)
  line L27 (62.6, 6) -> (65, 3.6)
  line L28 (65, 3.6) -> (65, 1.8)
  line L29 (65, 1.8) -> (63.2, 1.8)
  line L30 (63.2, 1.8) -> (65, 0)
  line L31 (65, 0) -> (70, 0)
  line L32 (70, 0) -> (70, 5)
  line L33 (70, 5) -> (68.2, 6.8)
  line L34 (68.2, 6.8) -> (68.2, 5)
  line L35 (68.2, 5) -> (66.4, 5)
  line L36 (66.4, 5) -> (64, 7.4)
  line L37 (64, 7.4) -> (64, 12.6)
  line L38 (64, 12.6) -> (66.4, 15)
  line L39 (66.4, 15) -> (68.2, 15)
  line L40 (68.2, 15) -> (68.2, 13.2)
  line L41 (68.2, 13.2) -> (70, 15)
  line L42 (70, 15) -> (70, 25)
  line L43 (70, 25) -> (68.2, 26.8)
  line L44 (68.2, 26.8) -> (68.2, 25)
  line L45 (68.2, 25) -> (66.4, 25)
  line L46 (66.4, 25) -> (64, 27.4)
  line L47 (64, 27.4) -> (64, 32.6)
  line L48 (64, 32.6) -> (66.4, 35)
  line L49 (66.4, 35) -> (68.2, 35)
  line L50 (68.2, 35) -> (68.2, 33.2)
  line L51 (68.2, 33.2) -> (70, 35)
  line L52 (70, 35) -> (70, 45)
  line L53 (70, 45) -> (68.2, 46.8)
  line L54 (68.2, 46.8) -> (68.2, 45)
  line L55 (68.2, 45) -> (66.4, 45)
  line L56 (66.4, 45) -> (64, 47.4)
  line L57 (64, 47.4) -> (64, 52.6)
  line L58 (64, 52.6) -> (66.4, 55)
  line L59 (66.4, 55) -> (68.2, 55)
  line L60 (68.2, 55) -> (68.2, 53.2)
  line L61 (68.2, 53.2) -> (70, 55)
  line L62 (70, 55) -> (70, 60)
  line L63 (70, 60) -> (65, 60)
  line L64 (65, 60) -> (63.2, 58.2)
  line L65 (63.2, 58.2) -> (65, 58.2)
  line L66 (65, 58.2) -> (65, 56.4)
  line L67 (65, 56.4) -> (62.6, 54)
  line L68 (62.6, 54) -> (57.4, 54)
  line L69 (57.4, 54) -> (55, 56.4)
  line L70 (55, 56.4) -> (55, 58.2)
  line L71 (55, 58.2) -> (56.8, 58.2)
  line L72 (56.8, 58.2) -> (55, 60)
  line L73 (55, 60) -> (50, 60)
  line L74 (50, 60) -> (50, 55)
  line L75 (50, 55) -> (51.8, 53.2)
  line L76 (51.8, 53.2) -> (51.8, 55)
  line L77 (51.8, 55) -> (53.6, 55)
  line L78 (53.6, 55) -> (56, 52.6)
  line L79 (56, 52.6) -> (56, 47.4)
  line L80 (56, 47.4) -> (53.6, 45)
  line L81 (53.6, 45) -> (51.8, 45)
  line L82 (51.8, 45) -> (51.8, 46.8)
  line L83 (51.8, 46.8) -> (50, 45)
  circle A0 centre (60, 50) radius 2.5
  line L84 (51.8, 40) -> (51.8, 43)
  line L85 (51.8, 43) -> (54.4, 43)
  line L86 (54.4, 43) -> (55, 43.6)
  line L87 (55, 43.6) -> (57.4, 46)
  line L88 (57.4, 46) -> (62.6, 46)
  line L89 (62.6, 46) -> (65.6, 43)
  line L90 (65.6, 43) -> (68.2, 43)
  line L91 (68.2, 43) -> (68.2, 40)
  line L92 (68.2, 40) -> (65, 40)
  line L93 (65, 40) -> (63.2, 38.2)
  line L94 (63.2, 38.2) -> (65, 38.2)
  line L95 (65, 38.2) -> (65, 36.4)
  line L96 (65, 36.4) -> (62.6, 34)
  line L97 (62.6, 34) -> (57.4, 34)
  line L98 (57.4, 34) -> (55, 36.4)
  line L99 (55, 36.4) -> (55, 38.2)
  line L100 (55, 38.2) -> (56.8, 38.2)
  line L101 (56.8, 38.2) -> (55, 40)
  line L102 (55, 40) -> (51.8, 40)
  circle A1 centre (60, 30) radius 2.5
  circle A2 centre (60, 10) radius 2.5
  line L103 (55, 23.6) -> (57.4, 26)
  line L104 (57.4, 26) -> (62.6, 26)
  line L105 (62.6, 26) -> (65, 23.6)
  line L106 (65, 23.6) -> (65, 21.8)
  line L107 (65, 21.8) -> (63.2, 21.8)
  line L108 (63.2, 21.8) -> (65, 20)
  line L109 (65, 20) -> (68.2, 20)
  line L110 (68.2, 20) -> (68.2, 17)
  line L111 (68.2, 17) -> (65.6, 17)
  line L112 (65.6, 17) -> (62.6, 14)
  line L113 (62.6, 14) -> (57.4, 14)
  line L114 (57.4, 14) -> (55, 16.4)
  line L115 (55, 16.4) -> (54.4, 17)
  line L116 (54.4, 17) -> (51.8, 17)
  line L117 (51.8, 17) -> (51.8, 20)
  line L118 (51.8, 20) -> (55, 20)
  line L119 (55, 20) -> (56.8, 21.8)
  line L120 (56.8, 21.8) -> (55, 21.8)
  line L121 (55, 21.8) -> (55, 23.6)
  line L122 (68.2, 20) -> (68.2, 23)
  line L123 (68.2, 23) -> (65.6, 23)
  line L124 (65.6, 23) -> (65, 23.6)
  line L125 (51.8, 20) -> (51.8, 23)
  line L126 (51.8, 23) -> (54.4, 23)
  line L127 (54.4, 23) -> (55, 23.6)
  line L128 (51.8, 40) -> (51.8, 37)
  line L129 (51.8, 37) -> (54.4, 37)
  line L130 (54.4, 37) -> (55, 36.4)
  line L131 (68.2, 40) -> (68.2, 37)
  line L132 (68.2, 37) -> (65.6, 37)
  line L133 (65.6, 37) -> (64.6866, 36.0866)
  dimension "d36" = 3
  dimension "d37" = 3
  dimension "d38" = 3
  dimension "d39" = 3
  constraint coincident L109.end L110.start
  constraint perpendicular L45 L122
  constraint perpendicular L122 L123
  constraint coincident L105.end L106.start
  constraint coincident L117.end L118.start
  constraint perpendicular L118 L125
  constraint perpendicular L125 L126
  constraint coincident L103.start L121.end
  constraint coincident L84.start L102.end
  constraint perpendicular L102 L128
  constraint perpendicular L128 L129
  constraint coincident L98.end L99.start
  constraint coincident L91.end L92.start
  constraint perpendicular L92 L131
  constraint perpendicular L95 L132
  constraint coincident L96 L133.end
  measures "d36" distance of L109.end L122.end
  measures "d37" distance of L117.end L125.end
  measures "d38" distance of L84.start L128.end
  measures "d39" distance of L91.end L131.end
extrude "Extrusion5" cut sketch "Skizze5" against normal blind 100 contours L99 L100 L101 L102 L128 L129 L130 | L92 L93 L94 L95 L131 L132 L133 | L118 L119 L120 L121 L125 L126 L127 | L106 L107 L108 L109 L122 L123 L124 bodies 4
sketch "Skizze6" plane through (0, 0, 200) normal (0, 0, 1) x (1, 0, 0)
  line L0 (90, 40) -> (88.2, 38.2)
  line L1 (88.2, 38.2) -> (90, 38.2)
  line L2 (90, 38.2) -> (90, 36.4)
  line L3 (90, 36.4) -> (87.6, 34)
  line L4 (87.6, 34) -> (82.4, 34)
  line L5 (82.4, 34) -> (80, 36.4)
  line L6 (80, 36.4) -> (80, 38.2)
  line L7 (80, 38.2) -> (81.8, 38.2)
  line L8 (81.8, 38.2) -> (80, 40)
  line L9 (80, 40) -> (81.8, 41.8)
  line L10 (81.8, 41.8) -> (80, 41.8)
  line L11 (80, 41.8) -> (80, 43.6)
  line L12 (80, 43.6) -> (82.4, 46)
  line L13 (82.4, 46) -> (87.6, 46)
  line L14 (87.6, 46) -> (90, 43.6)
  line L15 (90, 43.6) -> (90, 41.8)
  line L16 (90, 41.8) -> (88.2, 41.8)
  line L17 (88.2, 41.8) -> (90, 40)
  circle A0 centre (85, 50) radius 2.5
  circle A1 centre (85, 70) radius 2.5
  line L18 (79.4, 63) -> (80, 63.6)
  line L19 (80, 63.6) -> (82.4, 66)
  line L20 (82.4, 66) -> (87.6, 66)
  line L21 (87.6, 66) -> (90.6, 63)
  line L22 (90.6, 63) -> (93.2, 63)
  line L23 (93.2, 63) -> (93.2, 57)
  line L24 (93.2, 57) -> (90.6, 57)
  line L25 (90.6, 57) -> (87.6, 54)
  line L26 (87.6, 54) -> (82.4, 54)
  line L27 (82.4, 54) -> (80, 56.4)
  line L28 (80, 56.4) -> (79.4, 57)
  line L29 (79.4, 57) -> (76.8, 57)
  line L30 (76.8, 57) -> (76.8, 63)
  line L31 (76.8, 63) -> (79.4, 63)
  line L32 (79.4, 23) -> (80, 23.6)
  line L33 (80, 23.6) -> (82.4, 26)
  line L34 (82.4, 26) -> (87.6, 26)
  line L35 (87.6, 26) -> (90.6, 23)
  line L36 (90.6, 23) -> (93.2, 23)
  line L37 (93.2, 23) -> (93.2, 17)
  line L38 (93.2, 17) -> (90.6, 17)
  line L39 (90.6, 17) -> (87.6, 14)
  line L40 (87.6, 14) -> (82.4, 14)
  line L41 (82.4, 14) -> (80, 16.4)
  line L42 (80, 16.4) -> (79.4, 17)
  line L43 (79.4, 17) -> (76.8, 17)
  line L44 (76.8, 17) -> (76.8, 23)
  line L45 (76.8, 23) -> (79.4, 23)
  circle A2 centre (85, 30) radius 2.5
  circle A3 centre (85, 10) radius 2.5
  line L46 (95, 35) -> (95, 45)
  line L47 (95, 45) -> (93.2, 46.8)
  line L48 (93.2, 46.8) -> (93.2, 45)
  line L49 (93.2, 45) -> (91.4, 45)
  line L50 (91.4, 45) -> (89, 47.4)
  line L51 (89, 47.4) -> (89, 52.6)
  line L52 (89, 52.6) -> (91.4, 55)
  line L53 (91.4, 55) -> (93.2, 55)
  line L54 (93.2, 55) -> (93.2, 53.2)
  line L55 (93.2, 53.2) -> (95, 55)
  line L56 (95, 55) -> (95, 65)
  line L57 (95, 65) -> (93.2, 66.8)
  line L58 (93.2, 66.8) -> (93.2, 65)
  line L59 (93.2, 65) -> (91.4, 65)
  line L60 (91.4, 65) -> (89, 67.4)
  line L61 (89, 67.4) -> (89, 72.6)
  line L62 (89, 72.6) -> (91.4, 75)
  line L63 (91.4, 75) -> (93.2, 75)
  line L64 (93.2, 75) -> (93.2, 73.2)
  line L65 (93.2, 73.2) -> (95, 75)
  line L66 (95, 75) -> (95, 80)
  line L67 (95, 80) -> (90, 80)
  line L68 (90, 80) -> (88.2, 78.2)
  line L69 (88.2, 78.2) -> (90, 78.2)
  line L70 (90, 78.2) -> (90, 76.4)
  line L71 (90, 76.4) -> (87.6, 74)
  line L72 (87.6, 74) -> (82.4, 74)
  line L73 (82.4, 74) -> (80, 76.4)
  line L74 (80, 76.4) -> (80, 78.2)
  line L75 (80, 78.2) -> (81.8, 78.2)
  line L76 (81.8, 78.2) -> (80, 80)
  line L77 (80, 80) -> (75, 80)
  line L78 (75, 80) -> (75, 75)
  line L79 (75, 75) -> (76.8, 73.2)
  line L80 (76.8, 73.2) -> (76.8, 75)
  line L81 (76.8, 75) -> (78.6, 75)
  line L82 (78.6, 75) -> (81, 72.6)
  line L83 (81, 72.6) -> (81, 67.4)
  line L84 (81, 67.4) -> (78.6, 65)
  line L85 (78.6, 65) -> (76.8, 65)
  line L86 (76.8, 65) -> (76.8, 66.8)
  line L87 (76.8, 66.8) -> (75, 65)
  line L88 (75, 65) -> (75, 55)
  line L89 (75, 55) -> (76.8, 53.2)
  line L90 (76.8, 53.2) -> (76.8, 55)
  line L91 (76.8, 55) -> (78.6, 55)
  line L92 (78.6, 55) -> (81, 52.6)
  line L93 (81, 52.6) -> (81, 47.4)
  line L94 (81, 47.4) -> (78.6, 45)
  line L95 (78.6, 45) -> (76.8, 45)
  line L96 (76.8, 45) -> (76.8, 46.8)
  line L97 (76.8, 46.8) -> (75, 45)
  line L98 (75, 45) -> (75, 35)
  line L99 (75, 35) -> (76.8, 33.2)
  line L100 (76.8, 33.2) -> (76.8, 35)
  line L101 (76.8, 35) -> (78.6, 35)
  line L102 (78.6, 35) -> (81, 32.6)
  line L103 (81, 32.6) -> (81, 27.4)
  line L104 (81, 27.4) -> (78.6, 25)
  line L105 (78.6, 25) -> (76.8, 25)
  line L106 (76.8, 25) -> (76.8, 26.8)
  line L107 (76.8, 26.8) -> (75, 25)
  line L108 (75, 25) -> (75, 15)
  line L109 (75, 15) -> (76.8, 13.2)
  line L110 (76.8, 13.2) -> (76.8, 15)
  line L111 (76.8, 15) -> (78.6, 15)
  line L112 (78.6, 15) -> (81, 12.6)
  line L113 (81, 12.6) -> (81, 7.4)
  line L114 (81, 7.4) -> (78.6, 5)
  line L115 (78.6, 5) -> (76.8, 5)
  line L116 (76.8, 5) -> (76.8, 6.8)
  line L117 (76.8, 6.8) -> (75, 5)
  line L118 (75, 5) -> (75, 0)
  line L119 (75, 0) -> (80, 0)
  line L120 (80, 0) -> (81.8, 1.8)
  line L121 (81.8, 1.8) -> (80, 1.8)
  line L122 (80, 1.8) -> (80, 3.6)
  line L123 (80, 3.6) -> (82.4, 6)
  line L124 (82.4, 6) -> (87.6, 6)
  line L125 (87.6, 6) -> (90, 3.6)
  line L126 (90, 3.6) -> (90, 1.8)
  line L127 (90, 1.8) -> (88.2, 1.8)
  line L128 (88.2, 1.8) -> (90, 0)
  line L129 (90, 0) -> (95, 0)
  line L130 (95, 0) -> (95, 5)
  line L131 (95, 5) -> (93.2, 6.8)
  line L132 (93.2, 6.8) -> (93.2, 5)
  line L133 (93.2, 5) -> (91.4, 5)
  line L134 (91.4, 5) -> (89, 7.4)
  line L135 (89, 7.4) -> (89, 12.6)
  line L136 (89, 12.6) -> (91.4, 15)
  line L137 (91.4, 15) -> (93.2, 15)
  line L138 (93.2, 15) -> (93.2, 13.2)
  line L139 (93.2, 13.2) -> (95, 15)
  line L140 (95, 15) -> (95, 25)
  line L141 (95, 25) -> (93.2, 26.8)
  line L142 (93.2, 26.8) -> (93.2, 25)
  line L143 (93.2, 25) -> (91.4, 25)
  line L144 (91.4, 25) -> (89, 27.4)
  line L145 (89, 27.4) -> (89, 32.6)
  line L146 (89, 32.6) -> (91.4, 35)
  line L147 (91.4, 35) -> (93.2, 35)
  line L148 (93.2, 35) -> (93.2, 33.2)
  line L149 (93.2, 33.2) -> (95, 35)
  line L150 (76.8, 45) -> (76.8, 43)
  line L151 (76.8, 43) -> (79.8, 43)
  line L152 (79.8, 43) -> (79.8, 37)
  line L153 (79.8, 37) -> (76.8, 37)
  line L154 (76.8, 37) -> (76.8, 43)
  line L155 (93.2, 45) -> (93.2, 43)
  line L156 (93.2, 43) -> (90.3325, 43)
  line L157 (90.3325, 43) -> (90.3325, 37)
  line L158 (90.3325, 37) -> (93.2, 37)
  line L159 (93.2, 37) -> (93.2, 43)
  line L160 (80, 36.4) -> (79.4, 37)
  line L161 (80, 43.6) -> (79.4, 43)
  line L162 (90, 43.6) -> (90.6, 43)
  line L163 (90, 36.4) -> (90.6, 37)
  dimension "d42" = 2
  dimension "d43" = 6
  dimension "d44" = 2
  dimension "d45" = 6
  constraint coincident L95.end L96.start
  constraint perpendicular L95 L150
  constraint horizontal L151
  constraint vertical L152
  constraint horizontal L153
  constraint vertical L154
  constraint coincident L48.end L49.start
  constraint perpendicular L49 L155
  constraint horizontal L156
  constraint vertical L157
  constraint horizontal L158
  constraint vertical L159
  constraint coincident L5.end L6.start
  constraint coincident L153 L160.end
  constraint parallel L5 L160
  constraint coincident L11.end L12.start
  constraint coincident L151 L161.end
  constraint perpendicular L160 L161
  constraint coincident L14.end L15.start
  constraint coincident L156 L162.end
  constraint perpendicular L161 L162
  constraint coincident L2.end L3.start
  constraint coincident L158 L163.end
  constraint perpendicular L162 L163
  measures "d42" distance of L95.end L150.end
  measures "d43" distance of L150.end L153.end
  measures "d44" distance of L48.end L155.end
  measures "d45" distance of L155.end L158.end
extrude "Extrusion6" cut sketch "Skizze6" against normal blind 100 contours L0 L1 L2 L15 L16 L17 L156 L157 L158 L162 L163 | L156 L157 L158 L159 | L6 L7 L8 L9 L10 L11 L151 L152 L153 L160 L161 | L151 L152 L153 L154 bodies 6
copy_body "Körper kopieren/einfügen7" bodies 1 2 4 6 makes body 8 makes body 9 makes body 10 makes body 11
move_body "Verschieben7" bodies 8 9 10 11 to x (1, 0, 0) y (0, 1, 0) z (0, 0, 1) at (100, 0, 0)
move_body "Move8" bodies 1 to x (1, 0, 0) y (0, 1, 0) z (0, 0, 1) at (-10, -10, 0)
delete_body "RemoveBody1" bodies 2
delete_body "RemoveBody2" bodies 4
delete_body "RemoveBody3" bodies 6
delete_body "RemoveBody4" bodies 8
delete_body "RemoveBody5" bodies 9
delete_body "RemoveBody6" bodies 11
delete_body "RemoveBody7" bodies 10
move_body "Move9" bodies 1 to x (1, 0, 0) y (0, 1, 0) z (0, 0, 1) at (0, 0, 0)
fillet "Fillet1" radius 0.5 4 edges at (-10, 10, 0) (10, 10, 0) (10, -10, 0) (-10, -10, 0) on bodies 1
move_body "Move10" bodies 1 to x (1, 0, 0) y (0, 1, 0) z (0, 0, 1) at (-10, 0, 0)
delete_face "DeleteFace1" 2 faces at (-0.329, 9.9698, -66.6667) (-0.329, -9.9698, -66.6667) on bodies 1
copy_body "CopyPasteBodies8" bodies 1 makes body 12
move_body "Move11" bodies 12 to x (-1, 0, 0) y (0, -1, 0) z (0, 0, 1) at (0, 0, 0)
combine "Combine4" operation add target body 1 tool bodies 12